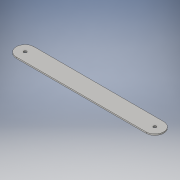
# Autodesk Inventor part: upper link
Saved by Autodesk Inventor 2016 (Build 200138000, 138)
## iProperties
Created: 2016-04-21
Part Number: upper link
Material: Generic
Document SubType Name: Modeling
Designer: Sam
Density: 1 g/cm^3
Appearance: Default
Author: Sam
Autodesk Inventor part; units mm, degrees
ref_plane "YZ Plane" through (0, 0, 0) normal (1, 0, 0) x (0, 1, 0)
ref_plane "XZ Plane" through (0, 0, 0) normal (0, 1, 0) x (-1, 0, 0)
ref_plane "XY Plane" through (0, 0, 0) normal (0, 0, 1) x (1, 0, 0)
sketch "Sketch1" plane through (0, 0, 0) normal (0, 1, 0) x (-1, 0, 0)
  line L0 (66, 0) -> (-66, 0) construction
  line L1 (66, 9) -> (-66, 9)
  line L2 (-66, -9) -> (66, -9)
  arc A0 (66, -9) -> (66, 9) centre (66, 0) ccw
  arc A1 (-66, 9) -> (-66, -9) centre (-66, 0) ccw
  point P0 (0, 0)
  dimension "d0" = 66
  dimension "d1" = 18
  constraints: 8 end point, 4 point on circle, 4 tangent, 2 centre point, 1 horizontal, 1 midpoint, 1 parallel
  measures "d0" distance of point (0, 0) L0.end
  measures "d1" diameter of A1
extrude "Extrusion1" add sketch "Sketch1" along normal blind 1.3
sketch "Sketch2" plane through (0, 1.3, 0) normal (0, 1, 0) x (1, 0, 0)
  arc A0 (-66, 9) -> (-66, -9) centre (-66, 0) ccw projected
  arc A1 (66, -9) -> (66, 9) centre (66, 0) ccw projected
  point P0 (0, 0)
  constraints: 2 coincident
hole "Hole1" at (-66, 1.3, 0) at (66, 1.3, 0) direction (0, -1, 0) diameter 3 end through all
thread "Thread1" size "M3x0.5" class "6H" standard "ANSI Metric M Profile" full length
thread "Thread2" size "M3x0.5" class "6H" standard "ANSI Metric M Profile" full length
body "Solid1"
